Autodesk Fusion 360 part; units mm, degrees
note: some values were not read from the file. Chosen so that the rebuilt part matches the saved one: which bodies a step acts on.
(part 2 of 4)
sketch "Sketch101" plane through (39, 814.3842, -118.7999) normal (1, 0, 0) x (0, 0, -1)
  line L0 (0, -84.3842) -> (0, 0) construction
  line L1 (0, 0) -> (18, 0) construction
  line L2 (0, 0) -> (2.1567, -2.1567) construction
  circle A0 centre (2.1567, -2.1567) radius 3.05
  dimension "d869" = 3.05
  constraint coincident L0.end L1.start
  constraint coincident L0.end A0
  measures "d869" distance of L0.end L2.end
sweep "Sweep8''''''''''" cut profiles "Sketch101" along 1 edges at (0, 77.5789, 44.7902) section 1 sketch seen with x (0, -0.5, 0.866025) y (0, 0.866025, 0.5) z (-1, 0, 0) at (-118.7999, -603.6986, -403.9712) on bodies 29 bodies 29 in component "Component''"
ref_plane "WorkPlane100" through (39, 904.3842, -174.7999) normal (1, 0, 0) x (0, 0, 1)
sketch "Sketch102" plane through (39, 904.3842, -174.7999) normal (1, 0, 0) x (0, 0, 1)
  line L0 (0, 0) -> (0, -84.3842) construction
  line L1 (0, 0) -> (18, 0) construction
  line L2 (0, 0) -> (2.1567, -2.1567) construction
  circle A0 centre (2.1567, -2.1567) radius 3.05
  dimension "d877" = 3.05
  constraint coincident L0.start L1.start
  constraint coincident L0.start A0
  measures "d877" distance of L0.start L2.end
sweep "Sweep5'''''''''''" cut profiles "Sketch102" along 1 edges at (0, 0, -179.5803) section 1 sketch seen with x (0, -1, 0) y (0, 0, -1) z (1, 0, 0) at (174.7999, 48, 724.8039) on bodies 28 bodies 28 in component "Component'"
ref_plane "WorkPlane101" through (57, 814.3842, -174.7999) normal (-1, 0, 0) x (0, 0, -1)
sketch "Sketch103" plane through (57, 814.3842, -174.7999) normal (-1, 0, 0) x (0, 0, -1)
  line L0 (0, 84.3842) -> (0, 0) construction
  line L1 (0, 0) -> (-18, 0) construction
  line L2 (0, 0) -> (-2.1567, 2.1567) construction
  circle A0 centre (-2.1567, 2.1567) radius 3.05
  dimension "d885" = 3.05
  constraint coincident L0.end L1.start
  constraint coincident L0.end A0
  measures "d885" distance of L0.end L2.end
sweep "Sweep6'''''''''''" cut profiles "Sketch103" along 1 edges at (0, 0, -89.5803) section 1 sketch seen with x (0, -1, 0) y (0, 0, -1) z (1, 0, 0) at (174.7999, 48, 724.8039) on bodies 28 bodies 28 in component "Component'"
ref_plane "WorkPlane102" through (57, 904.3842, -584.7999) normal (-1, 0, 0) x (0, 0, -1)
sketch "Sketch104" plane through (57, 904.3842, -584.7999) normal (-1, 0, 0) x (0, 0, -1)
  line L0 (0, 0) -> (0, -84.3842) construction
  line L1 (0, 0) -> (18, 0) construction
  line L2 (0, 0) -> (2.1567, -2.1567) construction
  circle A0 centre (2.1567, -2.1567) radius 3.05
  dimension "d893" = 3.05
  constraint coincident L0.start L1.start
  constraint coincident L0.start A0
  measures "d893" distance of L0.start L2.end
sweep "Sweep7'''''''''''" cut profiles "Sketch104" along 1 edges at (-410, 0, -179.5803) section 1 sketch seen with x (0, -1, 0) y (0, 0, -1) z (1, 0, 0) at (174.7999, 48, 724.8039) on bodies 28 bodies 28 in component "Component'"
ref_plane "WorkPlane103" through (39, 814.3842, -584.7999) normal (1, 0, 0) x (0, 0, 1)
sketch "Sketch105" plane through (39, 814.3842, -584.7999) normal (1, 0, 0) x (0, 0, 1)
  line L0 (0, 0) -> (0, 84.3842) construction
  line L1 (0, 0) -> (-18, 0) construction
  line L2 (0, 0) -> (-2.1567, 2.1567) construction
  circle A0 centre (-2.1567, 2.1567) radius 3.05
  dimension "d901" = 3.05
  constraint coincident L0.start L1.start
  constraint coincident L0.start A0
  measures "d901" distance of L0.start L2.end
sweep "Sweep8'''''''''''" cut profiles "Sketch105" along 1 edges at (-410, 0, -89.5803) section 1 sketch seen with x (0, -1, 0) y (0, 0, -1) z (1, 0, 0) at (174.7999, 48, 724.8039) on bodies 28 bodies 28 in component "Component'"
ref_plane "WorkPlane104" through (57, 1474.1009, -1297.9678) normal (-1, 0, 0) x (0, -0.866025, 0.5)
sketch "Sketch106" plane through (57, 1474.1009, -1297.9678) normal (-1, 0, 0) x (0, -0.866025, 0.5)
  line L0 (0, 0) -> (9.1, 15.7617) construction
  line L1 (43.4745, -25.1) -> (0, 0) construction
  line L2 (0, 0) -> (2.9461, 0.7894) construction
  circle A0 centre (2.9461, 0.7894) radius 3.05
  dimension "d909" = 3.05
  constraint coincident L0.start L1.end
  constraint coincident L0.start A0
  measures "d909" distance of L0.start L2.end
sweep "Sweep1" cut profiles "Sketch106" along 1 edges at (-27, 310.4558, -95.7894) section 1 sketch seen with x (1, 0, 0) y (0, 0.866025, 0.5) z (0, -0.5, 0.866025) at (-75, -1615.1369, 291.2332) on bodies 38 bodies 38 in component "Component'''''''''''"
ref_plane "WorkPlane105" through (57, 1474.1009, -1279.7678) normal (-1, 0, 0) x (0, -0.866025, 0.5)
sketch "Sketch107" plane through (57, 1474.1009, -1279.7678) normal (-1, 0, 0) x (0, -0.866025, 0.5)
  line L0 (0, 0) -> (-6.9433, -12.0262) construction
  line L1 (43.4745, -25.1) -> (0, 0) construction
  line L2 (0, 0) -> (0.7894, -2.9461) construction
  circle A0 centre (0.7894, -2.9461) radius 3.05
  dimension "d917" = 3.05
  constraint coincident L0.start L1.end
  constraint coincident L0.start A0
  measures "d917" distance of L0.start L2.end
sweep "Sweep2" cut profiles "Sketch107" along 1 edges at (-27, 301.3558, -80.0278) section 1 sketch seen with x (1, 0, 0) y (0, 0.866025, 0.5) z (0, -0.5, 0.866025) at (-75, -1615.1369, 291.2332) on bodies 38 bodies 38 in component "Component'''''''''''"
ref_plane "WorkPlane106" through (57, 1423.9009, -1297.9678) normal (-1, 0, 0) x (0, -0.866025, 0.5)
sketch "Sketch108" plane through (57, 1423.9009, -1297.9678) normal (-1, 0, 0) x (0, -0.866025, 0.5)
  line L0 (0, 0) -> (-39.739, 22.9433) construction
  line L1 (9.1, 15.7617) -> (0, 0) construction
  line L2 (0, 0) -> (-0.7894, 2.9461) construction
  circle A0 centre (-0.7894, 2.9461) radius 3.05
  dimension "d925" = 3.05
  constraint coincident L0.start L1.end
  constraint coincident L0.start A0
  measures "d925" distance of L0.start L2.end
sweep "Sweep3" cut profiles "Sketch108" along 1 edges at (-27, 266.9814, -120.8894) section 1 sketch seen with x (1, 0, 0) y (0, 0.866025, 0.5) z (0, -0.5, 0.866025) at (-75, -1615.1369, 291.2332) on bodies 38 bodies 38 in component "Component'''''''''''"
ref_plane "WorkPlane107" through (57, 1423.9009, -1279.7678) normal (-1, 0, 0) x (0, -0.866025, 0.5)
sketch "Sketch109" plane through (57, 1423.9009, -1279.7678) normal (-1, 0, 0) x (0, -0.866025, 0.5)
  line L0 (0, 0) -> (-6.9433, -12.0262) construction
  line L1 (-39.739, 22.9433) -> (0, 0) construction
  line L2 (0, 0) -> (-2.9461, -0.7894) construction
  circle A0 centre (-2.9461, -0.7894) radius 3.05
  dimension "d933" = 3.05
  constraint coincident L0.start L1.end
  constraint coincident L0.start A0
  measures "d933" distance of L0.start L2.end
sweep "Sweep4" cut profiles "Sketch109" along 1 edges at (-27, 257.8814, -105.1278) section 1 sketch seen with x (1, 0, 0) y (0, 0.866025, 0.5) z (0, -0.5, 0.866025) at (-75, -1615.1369, 291.2332) on bodies 38 bodies 38 in component "Component'''''''''''"
ref_plane "WorkPlane108" through (57, 1373.2979, -1327.1835) normal (-1, 0, 0) x (0, -0.866025, 0.5)
sketch "Sketch110" plane through (57, 1373.2979, -1327.1835) normal (-1, 0, 0) x (0, -0.866025, 0.5)
  line L0 (0, 0) -> (18.2, 0) construction
  line L1 (0, -50.2) -> (0, 0) construction
  line L2 (0, 0) -> (2.1567, -2.1567) construction
  circle A0 centre (2.1567, -2.1567) radius 3.05
  dimension "d941" = 3.05
  constraint coincident L0.start L1.end
  constraint coincident L0.start A0
  measures "d941" distance of L0.start L2.end
sweep "Sweep5''''''''''''" cut profiles "Sketch110" along 1 edges at (-27, 237.7657, -171.4924) section 1 sketch seen with x (1, 0, 0) y (0, 0.866025, 0.5) z (0, -0.5, 0.866025) at (-75, -1615.1369, 291.2332) on bodies 38 bodies 38 in component "Component'''''''''''"
ref_plane "WorkPlane109" through (57, 1357.5363, -1318.0835) normal (-1, 0, 0) x (0, -0.866025, 0.5)
sketch "Sketch111" plane through (57, 1357.5363, -1318.0835) normal (-1, 0, 0) x (0, -0.866025, 0.5)
  line L0 (0, 0) -> (0, -50.2) construction
  line L1 (-13.8866, 0) -> (0, 0) construction
  line L2 (0, 0) -> (-2.1567, -2.1567) construction
  circle A0 centre (-2.1567, -2.1567) radius 3.05
  dimension "d949" = 3.05
  constraint coincident L0.start L1.end
  constraint coincident L0.start A0
  measures "d949" distance of L0.start L2.end
sweep "Sweep6''''''''''''" cut profiles "Sketch111" along 1 edges at (-27, 219.5657, -171.4924) section 1 sketch seen with x (1, 0, 0) y (0, 0.866025, 0.5) z (0, -0.5, 0.866025) at (-75, -1615.1369, 291.2332) on bodies 38 bodies 38 in component "Component'''''''''''"
ref_plane "WorkPlane110" through (57, 1348.1979, -1370.6579) normal (-1, 0, 0) x (0, -0.866025, 0.5)
sketch "Sketch112" plane through (57, 1348.1979, -1370.6579) normal (-1, 0, 0) x (0, -0.866025, 0.5)
  line L0 (18.2, 0) -> (0, 0) construction
  line L1 (0, 0) -> (0, 45.8866) construction
  line L2 (0, 0) -> (2.1567, 2.1567) construction
  circle A0 centre (2.1567, 2.1567) radius 3.05
  dimension "d957" = 3.05
  constraint coincident L0.end L1.start
  constraint coincident L0.end A0
  measures "d957" distance of L0.end L2.end
sweep "Sweep7''''''''''''" cut profiles "Sketch112" along 1 edges at (-27, 237.7657, -221.6924) section 1 sketch seen with x (1, 0, 0) y (0, 0.866025, 0.5) z (0, -0.5, 0.866025) at (-75, -1615.1369, 291.2332) on bodies 38 bodies 38 in component "Component'''''''''''"
ref_plane "WorkPlane111" through (57, 1332.4363, -1361.5579) normal (-1, 0, 0) x (0, -0.866025, 0.5)
sketch "Sketch113" plane through (57, 1332.4363, -1361.5579) normal (-1, 0, 0) x (0, -0.866025, 0.5)
  line L0 (0, 0) -> (-13.8866, 0) construction
  line L1 (0, 45.8866) -> (0, 0) construction
  line L2 (0, 0) -> (-2.1567, 2.1567) construction
  circle A0 centre (-2.1567, 2.1567) radius 3.05
  dimension "d965" = 3.05
  constraint coincident L0.start L1.end
  constraint coincident L0.start A0
  measures "d965" distance of L0.start L2.end
sweep "Sweep8''''''''''''" cut profiles "Sketch113" along 1 edges at (-27, 219.5657, -221.6924) section 1 sketch seen with x (1, 0, 0) y (0, 0.866025, 0.5) z (0, -0.5, 0.866025) at (-75, -1615.1369, 291.2332) on bodies 38 bodies 38 in component "Component'''''''''''"
ref_plane "WorkPlane112" through (57, 1357.5363, -1259.6522) normal (-1, 0, 0) x (0, -0.866025, 0.5)
sketch "Sketch114" plane through (57, 1357.5363, -1259.6522) normal (-1, 0, 0) x (0, -0.866025, 0.5)
  line L0 (0, 0) -> (-9.1, 15.7617) construction
  line L1 (43.4745, 25.1) -> (0, 0) construction
  line L2 (0, 0) -> (0.7894, 2.9461) construction
  circle A0 centre (0.7894, 2.9461) radius 3.05
  dimension "d973" = 3.05
  constraint coincident L0.start L1.end
  constraint coincident L0.start A0
  measures "d973" distance of L0.start L2.end
sweep "Sweep9" cut profiles "Sketch114" along 1 edges at (-27, 190.3501, -120.8894) section 1 sketch seen with x (1, 0, 0) y (0, 0.866025, 0.5) z (0, -0.5, 0.866025) at (-75, -1615.1369, 291.2332) on bodies 38 bodies 38 in component "Component'''''''''''"
ref_plane "WorkPlane113" through (57, 1373.2979, -1250.5522) normal (-1, 0, 0) x (0, -0.866025, 0.5)
sketch "Sketch115" plane through (57, 1373.2979, -1250.5522) normal (-1, 0, 0) x (0, -0.866025, 0.5)
  line L0 (0, 0) -> (43.4745, 25.1) construction
  line L1 (6.9433, -12.0262) -> (0, 0) construction
  line L2 (0, 0) -> (2.9461, -0.7894) construction
  circle A0 centre (2.9461, -0.7894) radius 3.05
  dimension "d981" = 3.05
  constraint coincident L0.start L1.end
  constraint coincident L0.start A0
  measures "d981" distance of L0.start L2.end
sweep "Sweep10" cut profiles "Sketch115" along 1 edges at (-27, 199.4501, -105.1278) section 1 sketch seen with x (1, 0, 0) y (0, 0.866025, 0.5) z (0, -0.5, 0.866025) at (-75, -1615.1369, 291.2332) on bodies 38 bodies 38 in component "Component'''''''''''"
ref_plane "WorkPlane114" through (57, 1332.4363, -1216.1777) normal (-1, 0, 0) x (0, -0.866025, 0.5)
sketch "Sketch116" plane through (57, 1332.4363, -1216.1777) normal (-1, 0, 0) x (0, -0.866025, 0.5)
  line L0 (-9.1, 15.7617) -> (0, 0) construction
  line L1 (0, 0) -> (-39.739, -22.9433) construction
  line L2 (0, 0) -> (-2.9461, 0.7894) construction
  circle A0 centre (-2.9461, 0.7894) radius 3.05
  dimension "d989" = 3.05
  constraint coincident L0.end L1.start
  constraint coincident L0.end A0
  measures "d989" distance of L0.end L2.end
sweep "Sweep11" cut profiles "Sketch116" along 1 edges at (-27, 146.8756, -95.7894) section 1 sketch seen with x (1, 0, 0) y (0, 0.866025, 0.5) z (0, -0.5, 0.866025) at (-75, -1615.1369, 291.2332) on bodies 38 bodies 38 in component "Component'''''''''''"
ref_plane "WorkPlane115" through (57, 1348.1979, -1207.0777) normal (-1, 0, 0) x (0, -0.866025, 0.5)
sketch "Sketch117" plane through (57, 1348.1979, -1207.0777) normal (-1, 0, 0) x (0, -0.866025, 0.5)
  line L0 (0, 0) -> (6.9433, -12.0262) construction
  line L1 (-39.739, -22.9433) -> (0, 0) construction
  line L2 (0, 0) -> (-0.7894, -2.9461) construction
  circle A0 centre (-0.7894, -2.9461) radius 3.05
  dimension "d997" = 3.05
  constraint coincident L0.start L1.end
  constraint coincident L0.start A0
  measures "d997" distance of L0.start L2.end
sweep "Sweep12" cut profiles "Sketch117" along 1 edges at (-27, 155.9756, -80.0278) section 1 sketch seen with x (1, 0, 0) y (0, 0.866025, 0.5) z (0, -0.5, 0.866025) at (-75, -1615.1369, 291.2332) on bodies 38 bodies 38 in component "Component'''''''''''"
ref_plane "WorkPlane116" through (39, 1075.9239, -1204.8371) normal (1, 0, 0) x (0, 0, -1)
sketch "Sketch118" plane through (39, 1075.9239, -1204.8371) normal (1, 0, 0) x (0, 0, -1)
  line L0 (0, 0) -> (-9.1, 15.7617) construction
  line L1 (-78.1155, -45.1) -> (0, 0) construction
  line L2 (0, 0) -> (-2.9461, 0.7894) construction
  circle A0 centre (-2.9461, 0.7894) radius 3.05
  dimension "d1005" = 3.05
  constraint coincident L0.start L1.end
  constraint coincident L0.start A0
  measures "d1005" distance of L0.start L2.end
sweep "Sweep1'" cut profiles "Sketch118" along 1 edges at (9, 160.1577, 81.9593) section 1 sketch seen with x (1, 0, 0) y (0, 0, 1) z (0, -1, 0) at (-39, -1044.6793, -993.9645) on bodies 27 bodies 27 in component "Component"
ref_plane "WorkPlane117" through (39, 1091.6855, -1195.7371) normal (1, 0, 0) x (0, 0, -1)
sketch "Sketch119" plane through (39, 1091.6855, -1195.7371) normal (1, 0, 0) x (0, 0, -1)
  line L0 (0, 0) -> (-78.1155, -45.1) construction
  line L1 (6.9433, -12.0262) -> (0, 0) construction
  line L2 (0, 0) -> (-0.7894, -2.9461) construction
  circle A0 centre (-0.7894, -2.9461) radius 3.05
  dimension "d1013" = 3.05
  constraint coincident L0.start L1.end
  constraint coincident L0.start A0
  measures "d1013" distance of L0.start L2.end
sweep "Sweep2'" cut profiles "Sketch119" along 1 edges at (9, 151.0577, 97.721) section 1 sketch seen with x (1, 0, 0) y (0, 0, 1) z (0, -1, 0) at (-39, -1044.6793, -993.9645) on bodies 27 bodies 27 in component "Component"
ref_plane "WorkPlane118" through (39, 1030.8239, -1126.7216) normal (1, 0, 0) x (0, 0, -1)
sketch "Sketch120" plane through (39, 1030.8239, -1126.7216) normal (1, 0, 0) x (0, 0, -1)
  line L0 (-9.1, 15.7617) -> (0, 0) construction
  line L1 (0, 0) -> (74.38, 42.9433) construction
  line L2 (0, 0) -> (0.7894, 2.9461) construction
  circle A0 centre (0.7894, 2.9461) radius 3.05
  dimension "d1021" = 3.05
  constraint coincident L0.end L1.start
  constraint coincident L0.end A0
  measures "d1021" distance of L0.end L2.end
sweep "Sweep3'" cut profiles "Sketch120" along 1 edges at (9, 82.0423, 36.8593) section 1 sketch seen with x (1, 0, 0) y (0, 0, 1) z (0, -1, 0) at (-39, -1044.6793, -993.9645) on bodies 27 bodies 27 in component "Component"
ref_plane "WorkPlane119" through (39, 1046.5855, -1117.6216) normal (1, 0, 0) x (0, 0, -1)
sketch "Sketch121" plane through (39, 1046.5855, -1117.6216) normal (1, 0, 0) x (0, 0, -1)
  line L0 (0, 0) -> (6.9433, -12.0262) construction
  line L1 (74.38, 42.9433) -> (0, 0) construction
  line L2 (0, 0) -> (2.9461, -0.7894) construction
  circle A0 centre (2.9461, -0.7894) radius 3.05
  dimension "d1029" = 3.05
  constraint coincident L0.start L1.end
  constraint coincident L0.start A0
  measures "d1029" distance of L0.start L2.end
sweep "Sweep4'" cut profiles "Sketch121" along 1 edges at (9, 72.9423, 52.621) section 1 sketch seen with x (1, 0, 0) y (0, 0, 1) z (0, -1, 0) at (-39, -1044.6793, -993.9645) on bodies 27 bodies 27 in component "Component"
ref_plane "WorkPlane120" through (39, 904.4842, -1053.7793) normal (1, 0, 0) x (0, 0, -1)
sketch "Sketch122" plane through (39, 904.4842, -1053.7793) normal (1, 0, 0) x (0, 0, -1)
  line L0 (0, 0) -> (-18.2, 0) construction
  line L1 (0, -90.2) -> (0, 0) construction
  line L2 (0, 0) -> (-2.1567, -2.1567) construction
  circle A0 centre (-2.1567, -2.1567) radius 3.05
  dimension "d1037" = 3.05
  constraint coincident L0.start L1.end
  constraint coincident L0.start A0
  measures "d1037" distance of L0.start L2.end
sweep "Sweep5'''''''''''''" cut profiles "Sketch122" along 1 edges at (9, 9.1, -89.4803) section 1 sketch seen with x (1, 0, 0) y (0, 0, 1) z (0, -1, 0) at (-39, -1044.6793, -993.9645) on bodies 27 bodies 27 in component "Component"
ref_plane "WorkPlane121" through (39, 814.2842, -1053.7793) normal (1, 0, 0) x (0, 0, -1)
sketch "Sketch123" plane through (39, 814.2842, -1053.7793) normal (1, 0, 0) x (0, 0, -1)
  line L0 (0, 0) -> (0, 85.8866) construction
  line L1 (-18.2, 0) -> (0, 0) construction
  line L2 (0, 0) -> (-2.1567, 2.1567) construction
  circle A0 centre (-2.1567, 2.1567) radius 3.05
  dimension "d1045" = 3.05
  constraint coincident L0.start L1.end
  constraint coincident L0.start A0
  measures "d1045" distance of L0.start L2.end
sweep "Sweep6'''''''''''''" cut profiles "Sketch123" along 1 edges at (9, 9.1, -179.6803) section 1 sketch seen with x (1, 0, 0) y (0, 0, 1) z (0, -1, 0) at (-39, -1044.6793, -993.9645) on bodies 27 bodies 27 in component "Component"
ref_plane "WorkPlane122" through (39, 904.4842, -1035.5793) normal (1, 0, 0) x (0, 0, -1)
sketch "Sketch124" plane through (39, 904.4842, -1035.5793) normal (1, 0, 0) x (0, 0, -1)
  line L0 (0, 0) -> (0, -90.2) construction
  line L1 (13.8866, 0) -> (0, 0) construction
  line L2 (0, 0) -> (2.1567, -2.1567) construction
  circle A0 centre (2.1567, -2.1567) radius 3.05
  dimension "d1053" = 3.05
  constraint coincident L0.start L1.end
  constraint coincident L0.start A0
  measures "d1053" distance of L0.start L2.end
sweep "Sweep7'''''''''''''" cut profiles "Sketch124" along 1 edges at (9, -9.1, -89.4803) section 1 sketch seen with x (1, 0, 0) y (0, 0, 1) z (0, -1, 0) at (-39, -1044.6793, -993.9645) on bodies 27 bodies 27 in component "Component"
ref_plane "WorkPlane123" through (39, 814.2842, -1035.5793) normal (1, 0, 0) x (0, 0, -1)
sketch "Sketch125" plane through (39, 814.2842, -1035.5793) normal (1, 0, 0) x (0, 0, -1)
  line L0 (0, 0) -> (0, 85.8866) construction
  line L1 (13.8866, 0) -> (0, 0) construction
  line L2 (0, 0) -> (2.1567, 2.1567) construction
  circle A0 centre (2.1567, 2.1567) radius 3.05
  dimension "d1061" = 3.05
  constraint coincident L0.start L1.end
  constraint coincident L0.start A0
  measures "d1061" distance of L0.start L2.end
sweep "Sweep8'''''''''''''" cut profiles "Sketch125" along 1 edges at (9, -9.1, -179.6803) section 1 sketch seen with x (1, 0, 0) y (0, 0, 1) z (0, -1, 0) at (-39, -1044.6793, -993.9645) on bodies 27 bodies 27 in component "Component"
ref_plane "WorkPlane124" through (39, 1046.5855, -971.7371) normal (1, 0, 0) x (0, 0, -1)
sketch "Sketch126" plane through (39, 1046.5855, -971.7371) normal (1, 0, 0) x (0, 0, -1)
  line L0 (-9.1, -15.7617) -> (0, 0) construction
  line L1 (0, 0) -> (-78.1155, 45.1) construction
  line L2 (0, 0) -> (-2.9461, -0.7894) construction
  circle A0 centre (-2.9461, -0.7894) radius 3.05
  dimension "d1069" = 3.05
  constraint coincident L0.end L1.start
  constraint coincident L0.end A0
  measures "d1069" distance of L0.end L2.end
sweep "Sweep9'" cut profiles "Sketch126" along 1 edges at (9, -72.9423, 52.621) section 1 sketch seen with x (1, 0, 0) y (0, 0, 1) z (0, -1, 0) at (-39, -1044.6793, -993.9645) on bodies 27 bodies 27 in component "Component"
ref_plane "WorkPlane125" through (39, 1030.8239, -962.6371) normal (1, 0, 0) x (0, 0, -1)
sketch "Sketch127" plane through (39, 1030.8239, -962.6371) normal (1, 0, 0) x (0, 0, -1)
  line L0 (0, 0) -> (6.9433, 12.0262) construction
  line L1 (-78.1155, 45.1) -> (0, 0) construction
  line L2 (0, 0) -> (-0.7894, 2.9461) construction
  circle A0 centre (-0.7894, 2.9461) radius 3.05
  dimension "d1077" = 3.05
  constraint coincident L0.start L1.end
  constraint coincident L0.start A0
  measures "d1077" distance of L0.start L2.end
sweep "Sweep10'" cut profiles "Sketch127" along 1 edges at (9, -82.0423, 36.8593) section 1 sketch seen with x (1, 0, 0) y (0, 0, 1) z (0, -1, 0) at (-39, -1044.6793, -993.9645) on bodies 27 bodies 27 in component "Component"
ref_plane "WorkPlane126" through (39, 1091.6855, -893.6216) normal (1, 0, 0) x (0, 0, -1)
sketch "Sketch128" plane through (39, 1091.6855, -893.6216) normal (1, 0, 0) x (0, 0, -1)
  line L0 (0, 0) -> (-9.1, -15.7617) construction
  line L1 (74.38, -42.9433) -> (0, 0) construction
  line L2 (0, 0) -> (0.7894, -2.9461) construction
  circle A0 centre (0.7894, -2.9461) radius 3.05
  dimension "d1085" = 3.05
  constraint coincident L0.start L1.end
  constraint coincident L0.start A0
  measures "d1085" distance of L0.start L2.end
sweep "Sweep11'" cut profiles "Sketch128" along 1 edges at (9, -151.0577, 97.721) section 1 sketch seen with x (1, 0, 0) y (0, 0, 1) z (0, -1, 0) at (-39, -1044.6793, -993.9645) on bodies 27 bodies 27 in component "Component"
ref_plane "WorkPlane127" through (39, 1075.9239, -884.5216) normal (1, 0, 0) x (0, 0, -1)
sketch "Sketch129" plane through (39, 1075.9239, -884.5216) normal (1, 0, 0) x (0, 0, -1)
  line L0 (0, 0) -> (74.38, -42.9433) construction
  line L1 (6.9433, 12.0262) -> (0, 0) construction
  line L2 (0, 0) -> (2.9461, 0.7894) construction
  circle A0 centre (2.9461, 0.7894) radius 3.05
  dimension "d1093" = 3.05
  constraint coincident L0.start L1.end
  constraint coincident L0.start A0
  measures "d1093" distance of L0.start L2.end
sweep "Sweep12'" cut profiles "Sketch129" along 1 edges at (9, -160.1577, 81.9593) section 1 sketch seen with x (1, 0, 0) y (0, 0, 1) z (0, -1, 0) at (-39, -1044.6793, -993.9645) on bodies 27 bodies 27 in component "Component"
ref_plane "WorkPlane128" through (57, 1258.5761, -820.9975) normal (-1, 0, 0) x (0, 0, 1)
sketch "Sketch130" plane through (57, 1258.5761, -820.9975) normal (-1, 0, 0) x (0, 0, 1)
  line L0 (78.1155, -45.1) -> (0, 0) construction
  line L1 (0, 0) -> (9.1, 15.7617) construction
  line L2 (0, 0) -> (2.9461, 0.7894) construction
  circle A0 centre (2.9461, 0.7894) radius 3.05
  dimension "d1101" = 3.05
  constraint coincident L0.end L1.start
  constraint coincident L0.end A0
  measures "d1101" distance of L0.end L2.end
sweep "Sweep1''" cut profiles "Sketch130" along 1 edges at (-419, 160.1577, 81.9593) section 1 sketch seen with x (1, 0, 0) y (0, 0, 1) z (0, -1, 0) at (-467, -660.8398, -1176.6167) on bodies 32 bodies 32 in component "Component'''''"
ref_plane "WorkPlane129" through (57, 1274.3378, -811.8975) normal (-1, 0, 0) x (0, 0, 1)
sketch "Sketch131" plane through (57, 1274.3378, -811.8975) normal (-1, 0, 0) x (0, 0, 1)
  line L0 (-6.9433, -12.0262) -> (0, 0) construction
  line L1 (0, 0) -> (78.1155, -45.1) construction
  line L2 (0, 0) -> (0.7894, -2.9461) construction
  circle A0 centre (0.7894, -2.9461) radius 3.05
  dimension "d1109" = 3.05
  constraint coincident L0.end L1.start
  constraint coincident L0.end A0
  measures "d1109" distance of L0.end L2.end
sweep "Sweep2''" cut profiles "Sketch131" along 1 edges at (-419, 151.0577, 97.721) section 1 sketch seen with x (1, 0, 0) y (0, 0, 1) z (0, -1, 0) at (-467, -660.8398, -1176.6167) on bodies 32 bodies 32 in component "Component'''''"
ref_plane "WorkPlane130" through (57, 1229.2378, -733.782) normal (-1, 0, 0) x (0, 0, 1)
sketch "Sketch132" plane through (57, 1229.2378, -733.782) normal (-1, 0, 0) x (0, 0, 1)
  line L0 (0, 0) -> (-9.1, -15.7617) construction
  line L1 (-74.38, 42.9433) -> (0, 0) construction
  line L2 (0, 0) -> (-2.9461, -0.7894) construction
  circle A0 centre (-2.9461, -0.7894) radius 3.05
  dimension "d1117" = 3.05
  constraint coincident L0.start L1.end
  constraint coincident L0.start A0
  measures "d1117" distance of L0.start L2.end
sweep "Sweep3''" cut profiles "Sketch132" along 1 edges at (-419, 72.9423, 52.621) section 1 sketch seen with x (1, 0, 0) y (0, 0, 1) z (0, -1, 0) at (-467, -660.8398, -1176.6167) on bodies 32 bodies 32 in component "Component'''''"
ref_plane "WorkPlane131" through (57, 1213.4761, -742.882) normal (-1, 0, 0) x (0, 0, 1)
sketch "Sketch133" plane through (57, 1213.4761, -742.882) normal (-1, 0, 0) x (0, 0, 1)
  line L0 (6.9433, 12.0262) -> (0, 0) construction
  line L1 (0, 0) -> (-74.38, 42.9433) construction
  line L2 (0, 0) -> (-0.7894, 2.9461) construction
  circle A0 centre (-0.7894, 2.9461) radius 3.05
  dimension "d1125" = 3.05
  constraint coincident L0.end L1.start
  constraint coincident L0.end A0
  measures "d1125" distance of L0.end L2.end
sweep "Sweep4''" cut profiles "Sketch133" along 1 edges at (-419, 82.0423, 36.8593) section 1 sketch seen with x (1, 0, 0) y (0, 0, 1) z (0, -1, 0) at (-467, -660.8398, -1176.6167) on bodies 32 bodies 32 in component "Component'''''"
ref_plane "WorkPlane132" through (57, 1087.1364, -669.9398) normal (-1, 0, 0) x (0, 0, 1)
sketch "Sketch134" plane through (57, 1087.1364, -669.9398) normal (-1, 0, 0) x (0, 0, 1)
  line L0 (0, -90.2) -> (0, 0) construction
  line L1 (0, 0) -> (18.2, 0) construction
  line L2 (0, 0) -> (2.1567, -2.1567) construction
  circle A0 centre (2.1567, -2.1567) radius 3.05
  dimension "d1133" = 3.05
  constraint coincident L0.end L1.start
  constraint coincident L0.end A0
  measures "d1133" distance of L0.end L2.end
sweep "Sweep5''''''''''''''" cut profiles "Sketch134" along 1 edges at (-419, 9.1, -89.4803) section 1 sketch seen with x (1, 0, 0) y (0, 0, 1) z (0, -1, 0) at (-467, -660.8398, -1176.6167) on bodies 32 bodies 32 in component "Component'''''"
ref_plane "WorkPlane133" through (57, 996.9364, -669.9398) normal (-1, 0, 0) x (0, 0, 1)
sketch "Sketch135" plane through (57, 996.9364, -669.9398) normal (-1, 0, 0) x (0, 0, 1)
  line L0 (18.2, 0) -> (0, 0) construction
  line L1 (0, 0) -> (0, 85.8866) construction
  line L2 (0, 0) -> (2.1567, 2.1567) construction
  circle A0 centre (2.1567, 2.1567) radius 3.05
  dimension "d1141" = 3.05
  constraint coincident L0.end L1.start
  constraint coincident L0.end A0
  measures "d1141" distance of L0.end L2.end
sweep "Sweep6''''''''''''''" cut profiles "Sketch135" along 1 edges at (-419, 9.1, -179.6803) section 1 sketch seen with x (1, 0, 0) y (0, 0, 1) z (0, -1, 0) at (-467, -660.8398, -1176.6167) on bodies 32 bodies 32 in component "Component'''''"
ref_plane "WorkPlane134" through (57, 1087.1364, -651.7398) normal (-1, 0, 0) x (0, 0, 1)
sketch "Sketch136" plane through (57, 1087.1364, -651.7398) normal (-1, 0, 0) x (0, 0, 1)
  line L0 (0, 0) -> (0, -90.2) construction
  line L1 (-13.8866, 0) -> (0, 0) construction
  line L2 (0, 0) -> (-2.1567, -2.1567) construction
  circle A0 centre (-2.1567, -2.1567) radius 3.05
  dimension "d1149" = 3.05
  constraint coincident L0.start L1.end
  constraint coincident L0.start A0
  measures "d1149" distance of L0.start L2.end
sweep "Sweep7''''''''''''''" cut profiles "Sketch136" along 1 edges at (-419, -9.1, -89.4803) section 1 sketch seen with x (1, 0, 0) y (0, 0, 1) z (0, -1, 0) at (-467, -660.8398, -1176.6167) on bodies 32 bodies 32 in component "Component'''''"
ref_plane "WorkPlane135" through (57, 996.9364, -651.7398) normal (-1, 0, 0) x (0, 0, 1)
sketch "Sketch137" plane through (57, 996.9364, -651.7398) normal (-1, 0, 0) x (0, 0, 1)
  line L0 (0, 85.8866) -> (0, 0) construction
  line L1 (0, 0) -> (-13.8866, 0) construction
  line L2 (0, 0) -> (-2.1567, 2.1567) construction
  circle A0 centre (-2.1567, 2.1567) radius 3.05
  dimension "d1157" = 3.05
  constraint coincident L0.end L1.start
  constraint coincident L0.end A0
  measures "d1157" distance of L0.end L2.end
sweep "Sweep8''''''''''''''" cut profiles "Sketch137" along 1 edges at (-419, -9.1, -179.6803) section 1 sketch seen with x (1, 0, 0) y (0, 0, 1) z (0, -1, 0) at (-467, -660.8398, -1176.6167) on bodies 32 bodies 32 in component "Component'''''"
ref_plane "WorkPlane136" through (57, 1229.2378, -587.8975) normal (-1, 0, 0) x (0, 0, 1)
sketch "Sketch138" plane through (57, 1229.2378, -587.8975) normal (-1, 0, 0) x (0, 0, 1)
  line L0 (9.1, -15.7617) -> (0, 0) construction
  line L1 (0, 0) -> (78.1155, 45.1) construction
  line L2 (0, 0) -> (2.9461, -0.7894) construction
  circle A0 centre (2.9461, -0.7894) radius 3.05
  dimension "d1165" = 3.05
  constraint coincident L0.end L1.start
  constraint coincident L0.end A0
  measures "d1165" distance of L0.end L2.end
sweep "Sweep9''" cut profiles "Sketch138" along 1 edges at (-419, -72.9423, 52.621) section 1 sketch seen with x (1, 0, 0) y (0, 0, 1) z (0, -1, 0) at (-467, -660.8398, -1176.6167) on bodies 32 bodies 32 in component "Component'''''"
ref_plane "WorkPlane137" through (57, 1213.4761, -578.7975) normal (-1, 0, 0) x (0, 0, 1)
sketch "Sketch139" plane through (57, 1213.4761, -578.7975) normal (-1, 0, 0) x (0, 0, 1)
  line L0 (0, 0) -> (-6.9433, 12.0262) construction
  line L1 (78.1155, 45.1) -> (0, 0) construction
  line L2 (0, 0) -> (0.7894, 2.9461) construction
  circle A0 centre (0.7894, 2.9461) radius 3.05
  dimension "d1173" = 3.05
  constraint coincident L0.start L1.end
  constraint coincident L0.start A0
  measures "d1173" distance of L0.start L2.end
sweep "Sweep10''" cut profiles "Sketch139" along 1 edges at (-419, -82.0423, 36.8593) section 1 sketch seen with x (1, 0, 0) y (0, 0, 1) z (0, -1, 0) at (-467, -660.8398, -1176.6167) on bodies 32 bodies 32 in component "Component'''''"
ref_plane "WorkPlane138" through (57, 1274.3378, -509.782) normal (-1, 0, 0) x (0, 0, 1)
sketch "Sketch140" plane through (57, 1274.3378, -509.782) normal (-1, 0, 0) x (0, 0, 1)
  line L0 (-74.38, -42.9433) -> (0, 0) construction
  line L1 (0, 0) -> (9.1, -15.7617) construction
  line L2 (0, 0) -> (-0.7894, -2.9461) construction
  circle A0 centre (-0.7894, -2.9461) radius 3.05
  dimension "d1181" = 3.05
  constraint coincident L0.end L1.start
  constraint coincident L0.end A0
  measures "d1181" distance of L0.end L2.end
sweep "Sweep11''" cut profiles "Sketch140" along 1 edges at (-419, -151.0577, 97.721) section 1 sketch seen with x (1, 0, 0) y (0, 0, 1) z (0, -1, 0) at (-467, -660.8398, -1176.6167) on bodies 32 bodies 32 in component "Component'''''"
ref_plane "WorkPlane139" through (57, 1258.5761, -500.682) normal (-1, 0, 0) x (0, 0, 1)
sketch "Sketch141" plane through (57, 1258.5761, -500.682) normal (-1, 0, 0) x (0, 0, 1)
  line L0 (-6.9433, 12.0262) -> (0, 0) construction
  line L1 (0, 0) -> (-74.38, -42.9433) construction
  line L2 (0, 0) -> (-2.9461, 0.7894) construction
  circle A0 centre (-2.9461, 0.7894) radius 3.05
  dimension "d1189" = 3.05
  constraint coincident L0.end L1.start
  constraint coincident L0.end A0
  measures "d1189" distance of L0.end L2.end
sweep "Sweep12''" cut profiles "Sketch141" along 1 edges at (-419, -160.1577, 81.9593) section 1 sketch seen with x (1, 0, 0) y (0, 0, 1) z (0, -1, 0) at (-467, -660.8398, -1176.6167) on bodies 32 bodies 32 in component "Component'''''"
ref_plane "WorkPlane140" through (39, 1168.4645, -442.0314) normal (1, 0, 0) x (0, -0.866025, 0.5)
sketch "Sketch142" plane through (39, 1168.4645, -442.0314) normal (1, 0, 0) x (0, -0.866025, 0.5)
  line L0 (-9.1, -15.7617) -> (0, 0) construction
  line L1 (0, 0) -> (43.4745, -25.1) construction
  line L2 (0, 0) -> (0.7894, -2.9461) construction
  circle A0 centre (0.7894, -2.9461) radius 3.05
  dimension "d1197" = 3.05
  constraint coincident L0.end L1.start
  constraint coincident L0.end A0
  measures "d1197" distance of L0.end L2.end
sweep "Sweep5'''''''''''''''" cut profiles "Sketch142" along 1 edges at (-419, 155.9756, -80.0278) section 1 sketch seen with x (1, 0, 0) y (0, -0.866025, -0.5) z (0, 0.5, -0.866025) at (-467, 1388.9112, 121.394) on bodies 40 bodies 40 in component "Component'''''''''''''"
ref_plane "WorkPlane141" through (39, 1184.2261, -432.9314) normal (1, 0, 0) x (0, -0.866025, 0.5)
sketch "Sketch143" plane through (39, 1184.2261, -432.9314) normal (1, 0, 0) x (0, -0.866025, 0.5)
  line L0 (43.4745, -25.1) -> (0, 0) construction
  line L1 (0, 0) -> (6.9433, 12.0262) construction
  line L2 (0, 0) -> (2.9461, 0.7894) construction
  circle A0 centre (2.9461, 0.7894) radius 3.05
  dimension "d1205" = 3.05
  constraint coincident L0.end L1.start
  constraint coincident L0.end A0
  measures "d1205" distance of L0.end L2.end
sweep "Sweep6'''''''''''''''" cut profiles "Sketch143" along 1 edges at (-419, 146.8756, -95.7894) section 1 sketch seen with x (1, 0, 0) y (0, -0.866025, -0.5) z (0, 0.5, -0.866025) at (-467, 1388.9112, 121.394) on bodies 40 bodies 40 in component "Component'''''''''''''"
ref_plane "WorkPlane142" through (39, 1143.3645, -398.557) normal (1, 0, 0) x (0, -0.866025, 0.5)
sketch "Sketch144" plane through (39, 1143.3645, -398.557) normal (1, 0, 0) x (0, -0.866025, 0.5)
  line L0 (0, 0) -> (-9.1, -15.7617) construction
  line L1 (-39.739, 22.9433) -> (0, 0) construction
  line L2 (0, 0) -> (-2.9461, -0.7894) construction
  circle A0 centre (-2.9461, -0.7894) radius 3.05
  dimension "d1213" = 3.05
  constraint coincident L0.start L1.end
  constraint coincident L0.start A0
  measures "d1213" distance of L0.start L2.end
sweep "Sweep7'''''''''''''''" cut profiles "Sketch144" along 1 edges at (-419, 199.4501, -105.1278) section 1 sketch seen with x (1, 0, 0) y (0, -0.866025, -0.5) z (0, 0.5, -0.866025) at (-467, 1388.9112, 121.394) on bodies 40 bodies 40 in component "Component'''''''''''''"
ref_plane "WorkPlane143" through (39, 1159.1261, -389.457) normal (1, 0, 0) x (0, -0.866025, 0.5)
sketch "Sketch145" plane through (39, 1159.1261, -389.457) normal (1, 0, 0) x (0, -0.866025, 0.5)
  line L0 (0, 0) -> (6.9433, 12.0262) construction
  line L1 (-39.739, 22.9433) -> (0, 0) construction
  line L2 (0, 0) -> (-0.7894, 2.9461) construction
  circle A0 centre (-0.7894, 2.9461) radius 3.05
  dimension "d1221" = 3.05
  constraint coincident L0.start L1.end
  constraint coincident L0.start A0
  measures "d1221" distance of L0.start L2.end
sweep "Sweep8'''''''''''''''" cut profiles "Sketch145" along 1 edges at (-419, 190.3501, -120.8894) section 1 sketch seen with x (1, 0, 0) y (0, -0.866025, -0.5) z (0, 0.5, -0.866025) at (-467, 1388.9112, 121.394) on bodies 40 bodies 40 in component "Component'''''''''''''"
ref_plane "WorkPlane144" through (39, 1159.1261, -331.0257) normal (1, 0, 0) x (0, -0.866025, 0.5)
sketch "Sketch146" plane through (39, 1159.1261, -331.0257) normal (1, 0, 0) x (0, -0.866025, 0.5)
  line L0 (0, 0) -> (18.2, 0) construction
  line L1 (0, -50.2) -> (0, 0) construction
  line L2 (0, 0) -> (2.1567, -2.1567) construction
  circle A0 centre (2.1567, -2.1567) radius 3.05
  dimension "d1229" = 3.05
  constraint coincident L0.start L1.end
  constraint coincident L0.start A0
  measures "d1229" distance of L0.start L2.end
sweep "Sweep9'''" cut profiles "Sketch146" along 1 edges at (-419, 219.5657, -171.4924) section 1 sketch seen with x (1, 0, 0) y (0, -0.866025, -0.5) z (0, 0.5, -0.866025) at (-467, 1388.9112, 121.394) on bodies 40 bodies 40 in component "Component'''''''''''''"
ref_plane "WorkPlane145" through (39, 1143.3645, -321.9257) normal (1, 0, 0) x (0, -0.866025, 0.5)
sketch "Sketch147" plane through (39, 1143.3645, -321.9257) normal (1, 0, 0) x (0, -0.866025, 0.5)
  line L0 (0, 0) -> (-13.8866, 0) construction
  line L1 (0, -50.2) -> (0, 0) construction
  line L2 (0, 0) -> (-2.1567, -2.1567) construction
  circle A0 centre (-2.1567, -2.1567) radius 3.05
  dimension "d1237" = 3.05
  constraint coincident L0.start L1.end
  constraint coincident L0.start A0
  measures "d1237" distance of L0.start L2.end
sweep "Sweep10'''" cut profiles "Sketch147" along 1 edges at (-419, 237.7657, -171.4924) section 1 sketch seen with x (1, 0, 0) y (0, -0.866025, -0.5) z (0, 0.5, -0.866025) at (-467, 1388.9112, 121.394) on bodies 40 bodies 40 in component "Component'''''''''''''"
ref_plane "WorkPlane146" through (39, 1184.2261, -287.5512) normal (1, 0, 0) x (0, -0.866025, 0.5)
sketch "Sketch148" plane through (39, 1184.2261, -287.5512) normal (1, 0, 0) x (0, -0.866025, 0.5)
  line L0 (18.2, 0) -> (0, 0) construction
  line L1 (0, 0) -> (0, 45.8866) construction
  line L2 (0, 0) -> (2.1567, 2.1567) construction
  circle A0 centre (2.1567, 2.1567) radius 3.05
  dimension "d1245" = 3.05
  constraint coincident L0.end L1.start
  constraint coincident L0.end A0
  measures "d1245" distance of L0.end L2.end
sweep "Sweep11'''" cut profiles "Sketch148" along 1 edges at (-419, 219.5657, -221.6924) section 1 sketch seen with x (1, 0, 0) y (0, -0.866025, -0.5) z (0, 0.5, -0.866025) at (-467, 1388.9112, 121.394) on bodies 40 bodies 40 in component "Component'''''''''''''"
ref_plane "WorkPlane147" through (39, 1168.4645, -278.4512) normal (1, 0, 0) x (0, -0.866025, 0.5)
sketch "Sketch149" plane through (39, 1168.4645, -278.4512) normal (1, 0, 0) x (0, -0.866025, 0.5)
  line L0 (0, 0) -> (0, 45.8866) construction
  line L1 (-13.8866, 0) -> (0, 0) construction
  line L2 (0, 0) -> (-2.1567, 2.1567) construction
  circle A0 centre (-2.1567, 2.1567) radius 3.05
  dimension "d1253" = 3.05
  constraint coincident L0.start L1.end
  constraint coincident L0.start A0
  measures "d1253" distance of L0.start L2.end
sweep "Sweep12'''" cut profiles "Sketch149" along 1 edges at (-419, 237.7657, -221.6924) section 1 sketch seen with x (1, 0, 0) y (0, -0.866025, -0.5) z (0, 0.5, -0.866025) at (-467, 1388.9112, 121.394) on bodies 40 bodies 40 in component "Component'''''''''''''"
ref_plane "WorkPlane148" through (39, 1092.7615, -369.3413) normal (1, 0, 0) x (0, -0.866025, 0.5)
sketch "Sketch150" plane through (39, 1092.7615, -369.3413) normal (1, 0, 0) x (0, -0.866025, 0.5)
  line L0 (9.1, -15.7617) -> (0, 0) construction
  line L1 (0, 0) -> (43.4745, 25.1) construction
  line L2 (0, 0) -> (2.9461, -0.7894) construction
  circle A0 centre (2.9461, -0.7894) radius 3.05
  dimension "d1261" = 3.05
  constraint coincident L0.end L1.start
  constraint coincident L0.end A0
  measures "d1261" distance of L0.end L2.end
sweep "Sweep13" cut profiles "Sketch150" along 1 edges at (-419, 257.8814, -105.1278) section 1 sketch seen with x (1, 0, 0) y (0, -0.866025, -0.5) z (0, 0.5, -0.866025) at (-467, 1388.9112, 121.394) on bodies 40 bodies 40 in component "Component'''''''''''''"
ref_plane "WorkPlane149" through (39, 1042.5615, -369.3413) normal (1, 0, 0) x (0, -0.866025, 0.5)
sketch "Sketch151" plane through (39, 1042.5615, -369.3413) normal (1, 0, 0) x (0, -0.866025, 0.5)
  line L0 (0, 0) -> (-39.739, -22.9433) construction
  line L1 (9.1, -15.7617) -> (0, 0) construction
  line L2 (0, 0) -> (-0.7894, -2.9461) construction
  circle A0 centre (-0.7894, -2.9461) radius 3.05
  dimension "d1269" = 3.05
  constraint coincident L0.start L1.end
  constraint coincident L0.start A0
  measures "d1269" distance of L0.start L2.end
sweep "Sweep14" cut profiles "Sketch151" along 1 edges at (-419, 301.3558, -80.0278) section 1 sketch seen with x (1, 0, 0) y (0, -0.866025, -0.5) z (0, 0.5, -0.866025) at (-467, 1388.9112, 121.394) on bodies 40 bodies 40 in component "Component'''''''''''''"
ref_plane "WorkPlane150" through (39, 1092.7615, -351.1413) normal (1, 0, 0) x (0, -0.866025, 0.5)
sketch "Sketch152" plane through (39, 1092.7615, -351.1413) normal (1, 0, 0) x (0, -0.866025, 0.5)
  line L0 (0, 0) -> (-6.9433, 12.0262) construction
  line L1 (43.4745, 25.1) -> (0, 0) construction
  line L2 (0, 0) -> (0.7894, 2.9461) construction
  circle A0 centre (0.7894, 2.9461) radius 3.05
  dimension "d1277" = 3.05
  constraint coincident L0.start L1.end
  constraint coincident L0.start A0
  measures "d1277" distance of L0.start L2.end
sweep "Sweep15" cut profiles "Sketch152" along 1 edges at (-419, 266.9814, -120.8894) section 1 sketch seen with x (1, 0, 0) y (0, -0.866025, -0.5) z (0, 0.5, -0.866025) at (-467, 1388.9112, 121.394) on bodies 40 bodies 40 in component "Component'''''''''''''"
ref_plane "WorkPlane151" through (39, 1042.5615, -351.1413) normal (1, 0, 0) x (0, -0.866025, 0.5)
sketch "Sketch153" plane through (39, 1042.5615, -351.1413) normal (1, 0, 0) x (0, -0.866025, 0.5)
  line L0 (0, 0) -> (-6.9433, 12.0262) construction
  line L1 (-39.739, -22.9433) -> (0, 0) construction
  line L2 (0, 0) -> (-2.9461, 0.7894) construction
  circle A0 centre (-2.9461, 0.7894) radius 3.05
  dimension "d1285" = 3.05
  constraint coincident L0.start L1.end
  constraint coincident L0.start A0
  measures "d1285" distance of L0.start L2.end
sweep "Sweep16" cut profiles "Sketch153" along 1 edges at (-419, 310.4558, -95.7894) section 1 sketch seen with x (1, 0, 0) y (0, -0.866025, -0.5) z (0, 0.5, -0.866025) at (-467, 1388.9112, 121.394) on bodies 40 bodies 40 in component "Component'''''''''''''"
ref_plane "WorkPlane152" through (39, 1188.0192, -188.6055) normal (1, 0, 0) x (0, 0, 1)
sketch "Sketch154" plane through (39, 1188.0192, -188.6055) normal (1, 0, 0) x (0, 0, 1)
  line L0 (0, 0) -> (9.1, 15.7617) construction
  line L1 (43.4745, -25.1) -> (0, 0) construction
  line L2 (0, 0) -> (2.9461, 0.7894) construction
  circle A0 centre (2.9461, 0.7894) radius 3.05
  dimension "d1293" = 3.05
  constraint coincident L0.start L1.end
  constraint coincident L0.start A0
  measures "d1293" distance of L0.start L2.end
sweep "Sweep1'''" cut profiles "Sketch154" along 1 edges at (-419, -310.3901, -95.2685) section 1 sketch seen with x (1, 0, 0) y (0, 0, -1) z (0, 1, 0) at (-467, -121.7847, 1092.7507) on bodies 33 bodies 33 in component "Component''''''"
ref_plane "WorkPlane153" through (39, 1172.2575, -179.5055) normal (1, 0, 0) x (0, 0, 1)
sketch "Sketch155" plane through (39, 1172.2575, -179.5055) normal (1, 0, 0) x (0, 0, 1)
  line L0 (0, 0) -> (43.4745, -25.1) construction
  line L1 (-6.9433, -12.0262) -> (0, 0) construction
  line L2 (0, 0) -> (0.7894, -2.9461) construction
  circle A0 centre (0.7894, -2.9461) radius 3.05
  dimension "d1301" = 3.05
  constraint coincident L0.start L1.end
  constraint coincident L0.start A0
  measures "d1301" distance of L0.start L2.end
sweep "Sweep2'''" cut profiles "Sketch155" along 1 edges at (-419, -301.2901, -79.5068) section 1 sketch seen with x (1, 0, 0) y (0, 0, -1) z (0, 1, 0) at (-467, -121.7847, 1092.7507) on bodies 33 bodies 33 in component "Component''''''"
ref_plane "WorkPlane154" through (39, 1213.1192, -145.131) normal (1, 0, 0) x (0, 0, 1)
sketch "Sketch156" plane through (39, 1213.1192, -145.131) normal (1, 0, 0) x (0, 0, 1)
  line L0 (0, 0) -> (-39.739, 22.9433) construction
  line L1 (9.1, 15.7617) -> (0, 0) construction
  line L2 (0, 0) -> (-0.7894, 2.9461) construction
  circle A0 centre (-0.7894, 2.9461) radius 3.05
  dimension "d1309" = 3.05
  constraint coincident L0.start L1.end
  constraint coincident L0.start A0
  measures "d1309" distance of L0.start L2.end
sweep "Sweep3'''" cut profiles "Sketch156" along 1 edges at (-419, -266.9156, -120.3685) section 1 sketch seen with x (1, 0, 0) y (0, 0, -1) z (0, 1, 0) at (-467, -121.7847, 1092.7507) on bodies 33 bodies 33 in component "Component''''''"
ref_plane "WorkPlane155" through (39, 1197.3575, -136.031) normal (1, 0, 0) x (0, 0, 1)
sketch "Sketch157" plane through (39, 1197.3575, -136.031) normal (1, 0, 0) x (0, 0, 1)
  line L0 (0, 0) -> (-39.739, 22.9433) construction
  line L1 (-6.9433, -12.0262) -> (0, 0) construction
  line L2 (0, 0) -> (-2.9461, -0.7894) construction
  circle A0 centre (-2.9461, -0.7894) radius 3.05
  dimension "d1317" = 3.05
  constraint coincident L0.start L1.end
  constraint coincident L0.start A0
  measures "d1317" distance of L0.start L2.end
sweep "Sweep4'''" cut profiles "Sketch157" along 1 edges at (-419, -257.8156, -104.6068) section 1 sketch seen with x (1, 0, 0) y (0, 0, -1) z (0, 1, 0) at (-467, -121.7847, 1092.7507) on bodies 33 bodies 33 in component "Component''''''"
ref_plane "WorkPlane156" through (39, 1313.9221, -115.9153) normal (1, 0, 0) x (0, 0, 1)
sketch "Sketch158" plane through (39, 1313.9221, -115.9153) normal (1, 0, 0) x (0, 0, 1)
  line L0 (0, 0) -> (0, 50.2) construction
  line L1 (18.2, 0) -> (0, 0) construction
  line L2 (0, 0) -> (2.1567, 2.1567) construction
  circle A0 centre (2.1567, 2.1567) radius 3.05
  dimension "d1325" = 3.05
  constraint coincident L0.start L1.end
  constraint coincident L0.start A0
  measures "d1325" distance of L0.start L2.end
sweep "Sweep5''''''''''''''''" cut profiles "Sketch158" along 1 edges at (-419, -237.7, -221.1715) section 1 sketch seen with x (1, 0, 0) y (0, 0, -1) z (0, 1, 0) at (-467, -121.7847, 1092.7507) on bodies 33 bodies 33 in component "Component''''''"
ref_plane "WorkPlane157" through (39, 1313.9221, -97.7153) normal (1, 0, 0) x (0, 0, 1)
sketch "Sketch159" plane through (39, 1313.9221, -97.7153) normal (1, 0, 0) x (0, 0, 1)
  line L0 (0, 0) -> (-13.8866, 0) construction
  line L1 (0, 50.2) -> (0, 0) construction
  line L2 (0, 0) -> (-2.1567, 2.1567) construction
  circle A0 centre (-2.1567, 2.1567) radius 3.05
  dimension "d1333" = 3.05
  constraint coincident L0.start L1.end
  constraint coincident L0.start A0
  measures "d1333" distance of L0.start L2.end
sweep "Sweep6''''''''''''''''" cut profiles "Sketch159" along 1 edges at (-419, -219.5, -221.1715) section 1 sketch seen with x (1, 0, 0) y (0, 0, -1) z (0, 1, 0) at (-467, -121.7847, 1092.7507) on bodies 33 bodies 33 in component "Component''''''"
ref_plane "WorkPlane158" through (39, 1263.7221, -115.9153) normal (1, 0, 0) x (0, 0, 1)
sketch "Sketch160" plane through (39, 1263.7221, -115.9153) normal (1, 0, 0) x (0, 0, 1)
  line L0 (0, 0) -> (0, -45.8866) construction
  line L1 (18.2, 0) -> (0, 0) construction
  line L2 (0, 0) -> (2.1567, -2.1567) construction
  circle A0 centre (2.1567, -2.1567) radius 3.05
  dimension "d1341" = 3.05
  constraint coincident L0.start L1.end
  constraint coincident L0.start A0
  measures "d1341" distance of L0.start L2.end
sweep "Sweep7''''''''''''''''" cut profiles "Sketch160" along 1 edges at (-419, -237.7, -170.9715) section 1 sketch seen with x (1, 0, 0) y (0, 0, -1) z (0, 1, 0) at (-467, -121.7847, 1092.7507) on bodies 33 bodies 33 in component "Component''''''"
ref_plane "WorkPlane159" through (39, 1263.7221, -97.7153) normal (1, 0, 0) x (0, 0, 1)
sketch "Sketch161" plane through (39, 1263.7221, -97.7153) normal (1, 0, 0) x (0, 0, 1)
  line L0 (0, 0) -> (0, -45.8866) construction
  line L1 (-13.8866, 0) -> (0, 0) construction
  line L2 (0, 0) -> (-2.1567, -2.1567) construction
  circle A0 centre (-2.1567, -2.1567) radius 3.05
  dimension "d1349" = 3.05
  constraint coincident L0.start L1.end
  constraint coincident L0.start A0
  measures "d1349" distance of L0.start L2.end
sweep "Sweep8''''''''''''''''" cut profiles "Sketch161" along 1 edges at (-419, -219.5, -170.9715) section 1 sketch seen with x (1, 0, 0) y (0, 0, -1) z (0, 1, 0) at (-467, -121.7847, 1092.7507) on bodies 33 bodies 33 in component "Component''''''"
ref_plane "WorkPlane160" through (39, 1197.3575, -77.5997) normal (1, 0, 0) x (0, 0, 1)
sketch "Sketch162" plane through (39, 1197.3575, -77.5997) normal (1, 0, 0) x (0, 0, 1)
  line L0 (0, 0) -> (43.4745, 25.1) construction
  line L1 (9.1, -15.7617) -> (0, 0) construction
  line L2 (0, 0) -> (2.9461, -0.7894) construction
  circle A0 centre (2.9461, -0.7894) radius 3.05
  dimension "d1357" = 3.05
  constraint coincident L0.start L1.end
  constraint coincident L0.start A0
  measures "d1357" distance of L0.start L2.end
sweep "Sweep9''''" cut profiles "Sketch162" along 1 edges at (-419, -199.3844, -104.6068) section 1 sketch seen with x (1, 0, 0) y (0, 0, -1) z (0, 1, 0) at (-467, -121.7847, 1092.7507) on bodies 33 bodies 33 in component "Component''''''"
ref_plane "WorkPlane161" through (39, 1213.1192, -68.4997) normal (1, 0, 0) x (0, 0, 1)
sketch "Sketch163" plane through (39, 1213.1192, -68.4997) normal (1, 0, 0) x (0, 0, 1)
  line L0 (43.4745, 25.1) -> (0, 0) construction
  line L1 (0, 0) -> (-6.9433, 12.0262) construction
  line L2 (0, 0) -> (0.7894, 2.9461) construction
  circle A0 centre (0.7894, 2.9461) radius 3.05
  dimension "d1365" = 3.05
  constraint coincident L0.end L1.start
  constraint coincident L0.end A0
  measures "d1365" distance of L0.end L2.end
sweep "Sweep10''''" cut profiles "Sketch163" along 1 edges at (-419, -190.2844, -120.3685) section 1 sketch seen with x (1, 0, 0) y (0, 0, -1) z (0, 1, 0) at (-467, -121.7847, 1092.7507) on bodies 33 bodies 33 in component "Component''''''"
ref_plane "WorkPlane162" through (39, 1172.2575, -34.1252) normal (1, 0, 0) x (0, 0, 1)
sketch "Sketch164" plane through (39, 1172.2575, -34.1252) normal (1, 0, 0) x (0, 0, 1)
  line L0 (0, 0) -> (9.1, -15.7617) construction
  line L1 (-39.739, -22.9433) -> (0, 0) construction
  line L2 (0, 0) -> (-0.7894, -2.9461) construction
  circle A0 centre (-0.7894, -2.9461) radius 3.05
  dimension "d1373" = 3.05
  constraint coincident L0.start L1.end
  constraint coincident L0.start A0
  measures "d1373" distance of L0.start L2.end
sweep "Sweep11''''" cut profiles "Sketch164" along 1 edges at (-419, -155.9099, -79.5068) section 1 sketch seen with x (1, 0, 0) y (0, 0, -1) z (0, 1, 0) at (-467, -121.7847, 1092.7507) on bodies 33 bodies 33 in component "Component''''''"